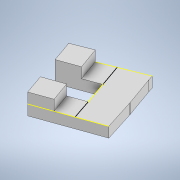
# Autodesk Inventor part: filendholder
Saved by Autodesk Inventor 2020 (Build 240168000, 168)
## iProperties
Created: 2019-07-05
Part Number: filendholder
Material: Generic
Document SubType Name: Modeling
Designer: ColinP
Density: 1 g/cm^3
Appearance: Default
Author: ColinP
Autodesk Inventor part; units mm, degrees
ref_plane "YZ Plane" through (0, 0, 0) normal (1, 0, 0) x (0, 1, 0)
ref_plane "XZ Plane" through (0, 0, 0) normal (0, 1, 0) x (-1, 0, 0)
ref_plane "XY Plane" through (0, 0, 0) normal (0, 0, 1) x (1, 0, 0)
sketch "Sketch1" plane through (0, 0, 0) normal (0, 1, 0) x (-1, 0, 0)
  line L0 (6.5186, 9.6083) -> (7.4793, 6.9251)
  line L1 (9.9904, -0.6602) -> (10.9974, -3.3263)
  line L2 (6.9989, 8.2667) -> (-2.8141, 4.7803)
  line L3 (10.4939, -1.9933) -> (0.6808, -5.4797)
  circle A0 centre (-12.8288, -4.5578) radius 1.5875
  circle A1 centre (-12.8288, -4.5578) radius 3.3389
  line L4 (-2.8141, 4.7803) -> (-12.8288, -4.5578)
  line L5 (-12.8288, -4.5578) -> (0.6808, -5.4797)
  line L6 (-2.8141, 4.7803) -> (-15.056, 0.431)
  line L7 (-12.8288, -4.5578) -> (-14.6522, 0.5745)
  line L8 (-14.6522, 0.5745) -> (-2.8141, 4.7803)
  line L9 (-12.8288, -4.5578) -> (-10.8725, -10.064)
  line L10 (0.6808, -5.4797) -> (-10.8725, -10.064)
  line L11 (10.4939, -1.9933) -> (11.3914, -4.3694)
  line L12 (11.3914, -4.3694) -> (9.5964, 0.3829)
  line L13 (9.5964, 0.3829) -> (-15.056, -8.4497)
  line L14 (-12.8288, -4.5578) -> (-15.975, -5.6756)
  line L15 (-15.9757, -5.6736) -> (-13.4484, -12.787)
  line L16 (-13.4484, -12.787) -> (-12.5471, -15.637)
  line L17 (11.3914, -4.3694) -> (-13.0447, -14.0634)
  line L18 (-15.9757, -5.6736) -> (-19.6824, 6.0465)
  line L19 (6.9989, 8.2667) -> (7.8493, 5.8733)
  line L20 (7.8493, 5.8733) -> (6.1486, 10.6602)
  line L21 (6.1486, 10.6602) -> (-18.3849, 1.9439)
  line L22 (7.8493, 5.8733) -> (-16.8521, -2.9027)
  line L23 (-2.8141, 4.7803) -> (0.6808, -5.4797)
  line L24 (-2.8141, 4.7803) -> (-3.6645, 7.1738)
  line L25 (0.6808, -5.4797) -> (1.6582, -8.2307)
  line L26 (-1.9951, 2.3758) -> (-16.8521, -2.9027)
  line L27 (-3.6645, 7.1738) -> (-18.3849, 1.9439)
  line L28 (-13.0447, -14.0634) -> (1.6582, -8.2307)
  line L29 (-0.1292, -3.1017) -> (-11.8537, -7.3024)
  line L30 (-0.1292, -3.1017) -> (1.6582, -8.2307)
  line L31 (-12.8288, -4.5578) -> (-9.6759, -3.4591)
  line L32 (-9.6759, -3.4591) -> (-6.8384, -11.6013)
  line L33 (-9.6759, -3.4591) -> (-12.2361, 4.1284)
  point P0 (0, 0)
  point P1 (-8.727, -6.1821)
  point P2 (-10.6118, -0.6856)
  point P3 (-16.045, -5.4546)
  point P4 (-15.9742, -5.6777)
  dimension "d0" = 10.414
  dimension "d1" = 10.414
  dimension "d2" = 12.2419
  dimension "d3" = 12.4297
  dimension "d4" = 5.1323
  dimension "d5" = 5.5062
  dimension "d6" = 13.6929
  dimension "d7" = 13.5096
  dimension "d8" = 2.54
  dimension "d9" = 5.08
  dimension "d10" = 2.54
  dimension "d11" = 5.08
  constraints: 68 end point, 17 point on line, 7 perpendicular, 3 parallel, 3 point on circle, 2 centre point, 2 collinear, 2 midpoint, 1 tangent
  measures "d0" distance of L2.start L2.end
  measures "d1" distance of L3.start L3.end
  measures "d2" horizontal distance of L2.end L6.end
  measures "d3" distance of L3.end L9.end
  measures "d4" vertical distance of L4.end L7.end
  measures "d5" vertical distance of L4.end L9.end
  measures "d6" distance of L2.end L4.end
  measures "d7" horizontal distance of L4.end L3.end
  measures "d8" distance of L3.start L11.end
  measures "d9" distance of L11.end L12.end
  measures "d10" distance of L2.start L19.end
  measures "d11" distance of L19.end L20.end
sketch "Sketch2" plane through (0, 0, 0) normal (0, 1, 0) x (-1, 0, 0)
  point P0 (0, 0)
extrude "Extrusion1" add sketch "Sketch1" along normal blind 2.54 contours L18 L22 A1 | L23 L5 L13 | L10 L32 L13 L5 | L25 L17 L32 L10 | L22 L4 L23 | L32 L17 L16 L15 L13 A1 L9 L10 | L10 L9 A1 L13 L32 | L32 L13 A1 L5 | L5 A1 L32 | L22 L33 L6 L4 | L6 L33 L21 L24 | L5 A0 L31 A1 | A1 L13 L9 A0 L5 | L31 A0 L4 A1 | A1 L4 L33 | A1 L9 L13 | L4 A1 L22 L33 | L22 A1 L7 L6 L33 | L6 L7 A1 L22 L18 L21 L33 | A1 L13 L9 | L5 L31 A0 | A0 L9 L5 | L4 A0 L7 L22 A1 | L31 L4 A0 | L13 A1 L14 A0 L9 | L22 L7 A1 | L13 L15 A1 | A0 L14 L9 | L7 A0 L4 | L14 A0 L7 | L7 L22 A1 | L7 A0 L14 A1 L22
sketch "Sketch3" plane through (0, 2.54, 0) normal (0, 1, 0) x (1, 0, 0)
  line L0 (8.727, 6.1821) -> (6.8384, 11.6013)
  line L1 (13.0447, 14.0634) -> (-1.6582, 8.2307) projected
  line L2 (10.6118, 0.6856) -> (12.2361, -4.1284)
  line L3 (3.6645, -7.1738) -> (18.3849, -1.9439) projected
  line L4 (8.727, 6.1821) -> (9.6759, 3.4591) projected
  line L5 (9.6759, 3.4591) -> (10.6118, 0.6856) projected
  point P0 (0, 0)
  constraints: 4 end point, 2 collinear, 2 point on line
sketch "Sketch4" plane through (0, 2.54, 0) normal (0, 1, 0) x (1, 0, 0)
  line L0 (2.8141, -4.7803) -> (3.6645, -7.1738) projected
  line L1 (1.9951, -2.3758) -> (3.6645, -7.1738)
  line L2 (3.6645, -7.1738) -> (8.4513, -5.4731)
  line L3 (3.6645, -7.1738) -> (18.3849, -1.9439) projected
  line L4 (8.4513, -5.4731) -> (6.7507, -0.6862)
  line L5 (10.6118, 0.6856) -> (1.9951, -2.3758) projected
  line L6 (-0.6808, 5.4797) -> (0.1292, 3.1017) projected
  line L7 (0.1292, 3.1017) -> (4.9115, 4.8151)
  line L8 (0.1292, 3.1017) -> (8.727, 6.1821) projected
  line L9 (4.9115, 4.8151) -> (3.0225, 10.0875)
  line L10 (13.0447, 14.0634) -> (-1.6582, 8.2307) projected
  line L11 (3.6645, -7.1738) -> (18.3849, -1.9439) projected
  line L12 (-1.6582, 8.2307) -> (-0.6808, 5.4797) projected
  line L13 (-0.6808, 5.4797) -> (-1.6582, 8.2307)
  point P0 (0, 0)
  dimension "d14" = 5.08
  dimension "d15" = 5.08
  constraints: 12 end point, 4 point on line, 3 perpendicular, 1 collinear
  measures "d14" distance of L0.end L2.end
  measures "d15" distance of L6.end L7.end
sketch "Sketch5" plane through (0, 2.54, 0) normal (0, 1, 0) x (1, 0, 0)
  point P0 (0, 0)
extrude "Extrusion2" add sketch "Sketch4" along normal blind 2.54
body "Solid1"
